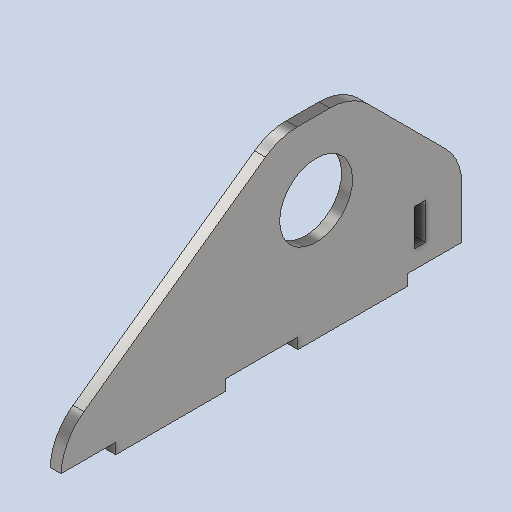
# Autodesk Inventor part: bottom_hinge_003
Saved by Autodesk Inventor 2025.2 (Build 292293000, 293)
## iProperties
Created: 2025-03-24
Part Number: bottom_hinge_003
Material: Stainless Steel
Document SubType Name: Sheet Metal
Designer: Caspe
Density: 8 g/cm^3
Sheet Metal Rule: Default_mm
Appearance: Semi-Polished
Flat Pattern Width: 10.0318 cm
Flat Pattern Length: 6.97486 cm
Flat Pattern Area: 69.9704 cm^2
Sheet Metal Width: 100,318 mm
Sheet Metal Length: 69,749 mm
Sheet Metal Area: 6997,045 mm^2
Author: Caspe
Autodesk Inventor part; units mm, degrees
ref_plane "YZ Plane" through (0, 0, 0) normal (1, 0, 0) x (0, 1, 0)
ref_plane "XZ Plane" through (0, 0, 0) normal (0, 1, 0) x (-1, 0, 0)
ref_plane "XY Plane" through (0, 0, 0) normal (0, 0, 1) x (1, 0, 0)
sketch "Sketch1" plane through (0, 0, 0) normal (1, 0, 0) x (0, 1, 0)
  line L0 (0, 0) -> (0, -120)
  line L1 (0, -120) -> (20, -120)
  line L2 (20, -120) -> (50, -90)
  line L3 (50, -90) -> (50, -70)
  line L4 (50, -70) -> (0, 0)
  line L5 (15, -107) -> (5, -107)
  line L6 (5, -107) -> (5, -110)
  line L7 (5, -110) -> (15, -110)
  line L8 (15, -110) -> (15, -107)
  line L9 (0, -105) -> (-3, -105)
  line L10 (-3, -105) -> (-3, -75)
  line L11 (-3, -75) -> (0, -75)
  line L12 (0, -75) -> (0, -105)
  line L13 (0, -55) -> (-3, -55)
  line L14 (-3, -55) -> (-3, -25)
  line L15 (-3, -25) -> (0, -25)
  line L16 (0, -25) -> (0, -55)
  line L17 (0, -10) -> (7.1429, -10)
  circle A0 centre (30, -80) radius 10
  line L18 (30, -80) -> (50, -80)
  point P0 (-1.5, -105)
  point P1 (-1.5, -75)
  point P2 (0, -25)
  point P3 (0, -75)
  dimension "d0" = 120
  dimension "d1" = 10
  dimension "d2" = 3
  dimension "d3" = 10
  dimension "d4" = 5
  dimension "d5" = 3
  dimension "d6" = 30
  dimension "d7" = 15
  dimension "d8" = 3
  dimension "d9" = 30
  dimension "d10" = 20
  dimension "d11" = 30
  dimension "d12" = 20
  dimension "d13" = 50
  dimension "d14" = 10
  dimension "d15" = 45
  dimension "d16" = 20
  dimension "d17" = 30
  dimension "d18" = 90
  measures "d0" distance of L0.start L0.end
  measures "d1" distance of L7.end L6.end
  measures "d2" distance of L6.end L5.end
  measures "d3" distance between parallel lines of L1 L7
  measures "d4" distance between parallel lines of L0 L6
  measures "d5" distance of L10.end L11.end
  measures "d6" distance of L9.end L10.end
  measures "d7" distance from line of L1 point (-1.5, -105)
  measures "d8" distance of L14.end L15.end
  measures "d9" distance of L13.end L14.end
  measures "d10" distance from line of point (-1.5, -75) L13
  measures "d11" distance from line of L2.end L1
  measures "d12" distance of L2.end L3.end
  measures "d13" distance between parallel lines of L12 L3
  measures "d14" distance from line of L0.start L17
  measures "d15" angle of L0 L2
  measures "d16" diameter of A0
  measures "d17" distance from line of L12 L18.start
  measures "d18" angle of L3 L18
extrude "Plate1" add sketch "Sketch1" along normal blind 3 contours L17 L4 L3 L2 L1 L0 | L0 L13 L14 L15 | L0 L9 L10 L11
fillet "Corner Round1" radius 15 4 edges at (1.5, 50, -70) (1.5, 50, -90) (1.5, 20, -120) (1.5, 7.1429, -10)
equation "\"d2\" = plate_thickness"
equation "\"d5\" = plate_thickness"
equation "\"d8\" = plate_thickness"
equation "\"d19\" = Thickness"
equation "\"Thickness\" = plate_thickness"
equation "\"BendRadius\" = Thickness"
equation "\"BendReliefWidth\" = Thickness"
equation "\"BendReliefDepth\" = 0.5 * Thickness"
equation "\"CornerReliefSize\" = 4 * Thickness"
equation "\"MinimumRemnant\" = 2 * Thickness"
equation "\"TransitionRadius\" = BendRadius"
equation "\"JacobiRadiusSize\" = BendRadius"
equation "\"GapSize\" = Thickness"
equation "\"A_width\" = 46"
equation "\"A_joint_diameter\" = 16"
equation "\"A_joint_tolerance\" = 3"
equation "\"l___________\" = 0"
equation "\"l__________\" = 0"
equation "\"l_________\" = 0"
equation "\"rivet_diameter\" = 3.35"
equation "\"plate_thickness\" = 3"
equation "\"l________\" = 0"
equation "\"A_B_spacing\" = 2"
equation "\"L_Piston_Bottom\" = 21"
equation "\"L_Piston_Top\" = 25"
equation "\"thin_plate\" = 1.5"
body "Solid1"
